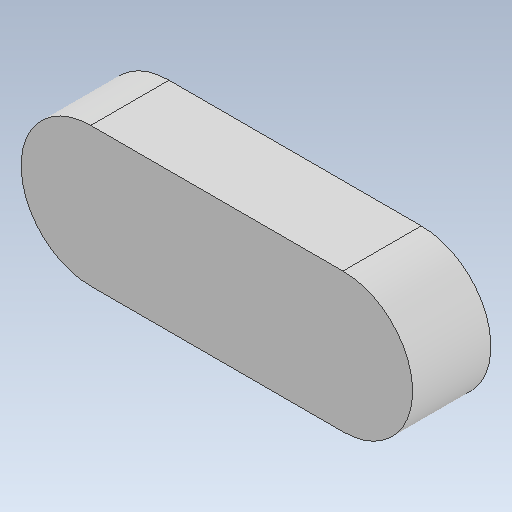
# Autodesk Inventor part: key5
Saved by Autodesk Inventor 2020 (Build 240168000, 168)
## iProperties
Created: 2021-06-15
Part Number: key5
Material: 常规
Document SubType Name: Modeling
Designer: dell
Density: 1 g/cm^3
Appearance: 默认
Author: dell
Autodesk Inventor part; units mm, degrees
ref_plane "YZ Plane" through (0, 0, 0) normal (1, 0, 0) x (0, 1, 0)
ref_plane "XZ Plane" through (0, 0, 0) normal (0, 1, 0) x (-1, 0, 0)
ref_plane "XY Plane" through (0, 0, 0) normal (0, 0, 1) x (1, 0, 0)
sketch "草图1" plane through (0, 0, 0) normal (0, 0, 1) x (1, 0, 0)
  line L0 (-23.5, 0) -> (34.5, 0) projected
  arc A0 (-23.5, 0) -> (-23.5, -32) centre (-23.5, -16) ccw projected
  line L1 (-23.5, -32) -> (34.5, -32) projected
  arc A1 (34.5, -32) -> (34.5, 0) centre (34.5, -16) ccw projected
  line L2 (34.5, -16) -> (-23.5, -16) construction
  line L3 (34.5, 0) -> (-23.5, 0)
  line L4 (-23.5, -32) -> (34.5, -32)
  arc A2 (34.5, -32) -> (34.5, 0) centre (34.5, -16) ccw
  arc A3 (-23.5, 0) -> (-23.5, -32) centre (-23.5, -16) ccw
  point P0 (0, 0)
  point P1 (5.5, -16)
  constraints: 8 end point, 4 point on circle, 4 tangent, 2 centre point, 1 concentric, 1 horizontal, 1 midpoint, 1 parallel
extrude "拉伸1" add sketch "草图1" along normal blind 18
